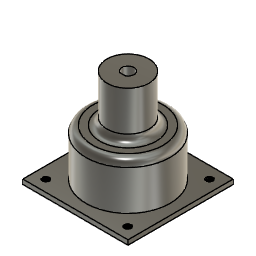
35mm_shaft_extension (Autodesk Fusion 360 design; units mm, degrees)
Autodesk Fusion 360 part; units mm, degrees
sketch "Sketch1" plane through (0, 0, 0) normal (0, 0, 1) x (1, 0, 0)
  line L0 (0, 0) -> (45, 0)
  line L1 (45, 0) -> (45, 45)
  line L2 (45, 45) -> (0, 45)
  line L3 (0, 45) -> (0, 0)
  dimension "d1" = 45
  dimension "d2" = 45
  constraint horizontal L0
  constraint vertical L1
  constraint horizontal L2
  constraint vertical L3
  constraint coincident L0.start L3.end
  measures "d1" distance of L0.start L0.end
  measures "d2" distance of L0.start L2.end
extrude "Extrude1" add sketch "Sketch1" along normal blind 2
sketch "Sketch2" plane through (0, 0, 2) normal (0, 0, 1) x (-1, 0, 0)
  line L0 (0, -45) -> (0, 0)
  line L1 (0, 0) -> (-45, 0)
  line L2 (-45, 0) -> (-45, -45)
  line L3 (-45, -45) -> (0, -45)
  line L4 (-40, -5) -> (-40, -40) construction
  line L5 (-40, -40) -> (-5, -40) construction
  line L6 (-5, -40) -> (-5, -5) construction
  line L7 (-5, -5) -> (-40, -5) construction
  circle A0 centre (-5, -40) radius 1.5
  circle A1 centre (-40, -40) radius 1.5
  circle A2 centre (-5, -5) radius 1.5
  circle A3 centre (-40, -5) radius 1.5
  dimension "d5" = -5
  dimension "d6" = 3
  dimension "d7" = 3
  dimension "d8" = 3
  dimension "d9" = 3
  constraint coincident L5.end L6.start
  constraint coincident L4.end L5.start
  constraint coincident L6.end L7.start
  constraint coincident L4.start L7.end
  measures "d6" diameter of A0
  measures "d7" diameter of A1
  measures "d8" diameter of A2
  measures "d9" diameter of A3
hole "Hole1" at (5, 40, 2) at (40, 40, 2) at (40, 5, 2) at (5, 5, 2) direction (0, 0, -1) diameter 2.529 depth 2 tip angle 118
thread "Thread1" "ISO Metric profile 3.0 M3x0.5 M3x0.5 6H" major diameter 3.086 minor diameter 2.529 pitch 0.5 angle 60 modelled right hand crest width 0.1368 on face at (3.7359, 40.0315, 1.3333) crest through (6.2645, 40, 1.875) on face at (5.1259, 3.7418, 1.3333) crest through (6.2645, 5, 1.875) on face at (40.8128, 40.9687, 1.3333) crest through (41.2645, 40, 1.875) on face at (40.1259, 6.2582, 1.3333) crest through (41.2645, 5, 1.875)
sketch "Sketch3" plane through (0, 0, 2) normal (0, 0, 1) x (-1, 0, 0)
  spline S0 degree 3 poles (-40.9581, -5.8252) (-41.0802, -5.7112) (-41.1784, -5.574) (-41.3207, -5.264) (-41.3611, -5.093) (-41.3757, -4.7382) (-41.3471, -4.5577) (-41.2212, -4.2109) (-41.1226, -4.0488) (-40.9156, -3.8208) (-40.8244, -3.7423) (-40.6232, -3.6071) (-40.5136, -3.5514) (-40.3985, -3.5094) knots 0 0 0 0 0.050111 0.050111 0.102261 0.102261 0.15645 0.15645 0.212677 0.212677 0.24852 0.24852 0.285143 0.285143 0.285143 0.285143
  arc A0 (-39.6015, -3.5094) -> (-40.3985, -3.5094) centre (-40, -5) ccw
  spline S1 degree 3 poles (-39.6015, -3.5094) (-39.4166, -3.5769) (-39.2465, -3.6793) (-38.9611, -3.9399) (-38.8468, -4.0935) (-38.6876, -4.4304) (-38.6419, -4.6092) (-38.6233, -4.9674) (-38.648, -5.1432) (-38.741, -5.4082) (-38.7875, -5.5028) (-38.901, -5.6765) (-38.967, -5.7553) (-39.0419, -5.8252) knots 0 0 0 0 0.059039 0.059039 0.116033 0.116033 0.170983 0.170983 0.223888 0.223888 0.255505 0.255505 0.286347 0.286347 0.286347 0.286347
  arc A1 (-40.9581, -5.8252) -> (-39.0419, -5.8252) centre (-40, -5) ccw
  spline S2 degree 3 poles (-5.9581, -40.8252) (-6.0802, -40.7112) (-6.1784, -40.574) (-6.3207, -40.264) (-6.3611, -40.093) (-6.3757, -39.7382) (-6.3471, -39.5577) (-6.2212, -39.2109) (-6.1226, -39.0488) (-5.9156, -38.8208) (-5.8244, -38.7423) (-5.6232, -38.6071) (-5.5136, -38.5514) (-5.3985, -38.5094) knots 0 0 0 0 0.050111 0.050111 0.102261 0.102261 0.15645 0.15645 0.212677 0.212677 0.24852 0.24852 0.285143 0.285143 0.285143 0.285143
  arc A2 (-4.6015, -38.5094) -> (-5.3985, -38.5094) centre (-5, -40) ccw
  spline S3 degree 3 poles (-4.6015, -38.5094) (-4.4166, -38.5769) (-4.2465, -38.6793) (-3.9611, -38.9399) (-3.8468, -39.0935) (-3.6876, -39.4304) (-3.6419, -39.6092) (-3.6233, -39.9674) (-3.648, -40.1432) (-3.741, -40.4082) (-3.7875, -40.5028) (-3.901, -40.6765) (-3.967, -40.7553) (-4.0419, -40.8252) knots 0 0 0 0 0.059039 0.059039 0.116033 0.116033 0.170983 0.170983 0.223888 0.223888 0.255505 0.255505 0.286347 0.286347 0.286347 0.286347
  arc A3 (-5.9581, -40.8252) -> (-4.0419, -40.8252) centre (-5, -40) ccw
  spline S4 degree 3 poles (-40.9581, -40.8252) (-41.0802, -40.7112) (-41.1784, -40.574) (-41.3207, -40.264) (-41.3611, -40.093) (-41.3757, -39.7382) (-41.3471, -39.5577) (-41.2212, -39.2109) (-41.1226, -39.0488) (-40.9156, -38.8208) (-40.8244, -38.7423) (-40.6232, -38.6071) (-40.5136, -38.5514) (-40.3985, -38.5094) knots 0 0 0 0 0.050111 0.050111 0.102261 0.102261 0.15645 0.15645 0.212677 0.212677 0.24852 0.24852 0.285143 0.285143 0.285143 0.285143
  arc A4 (-39.6015, -38.5094) -> (-40.3985, -38.5094) centre (-40, -40) ccw
  spline S5 degree 3 poles (-39.6015, -38.5094) (-39.4166, -38.5769) (-39.2465, -38.6793) (-38.9611, -38.9399) (-38.8468, -39.0935) (-38.6876, -39.4304) (-38.6419, -39.6092) (-38.6233, -39.9674) (-38.648, -40.1432) (-38.741, -40.4082) (-38.7875, -40.5028) (-38.901, -40.6765) (-38.967, -40.7553) (-39.0419, -40.8252) knots 0 0 0 0 0.059039 0.059039 0.116033 0.116033 0.170983 0.170983 0.223888 0.223888 0.255505 0.255505 0.286347 0.286347 0.286347 0.286347
  arc A5 (-40.9581, -40.8252) -> (-39.0419, -40.8252) centre (-40, -40) ccw
  spline S6 degree 3 poles (-5.9581, -5.8252) (-6.0802, -5.7112) (-6.1784, -5.574) (-6.3207, -5.264) (-6.3611, -5.093) (-6.3757, -4.7382) (-6.3471, -4.5577) (-6.2212, -4.2109) (-6.1226, -4.0488) (-5.9156, -3.8208) (-5.8244, -3.7423) (-5.6232, -3.6071) (-5.5136, -3.5514) (-5.3985, -3.5094) knots 0 0 0 0 0.050111 0.050111 0.102261 0.102261 0.15645 0.15645 0.212677 0.212677 0.24852 0.24852 0.285143 0.285143 0.285143 0.285143
  arc A6 (-4.6015, -3.5094) -> (-5.3985, -3.5094) centre (-5, -5) ccw
  spline S7 degree 3 poles (-4.6015, -3.5094) (-4.4166, -3.5769) (-4.2465, -3.6793) (-3.9611, -3.9399) (-3.8468, -4.0935) (-3.6876, -4.4304) (-3.6419, -4.6092) (-3.6233, -4.9674) (-3.648, -5.1432) (-3.741, -5.4082) (-3.7875, -5.5028) (-3.901, -5.6765) (-3.967, -5.7553) (-4.0419, -5.8252) knots 0 0 0 0 0.059039 0.059039 0.116033 0.116033 0.170983 0.170983 0.223888 0.223888 0.255505 0.255505 0.286347 0.286347 0.286347 0.286347
  arc A7 (-5.9581, -5.8252) -> (-4.0419, -5.8252) centre (-5, -5) ccw
  line L0 (0, -45) -> (0, 0)
  line L1 (0, 0) -> (-45, 0)
  line L2 (-45, 0) -> (-45, -45)
  line L3 (-45, -45) -> (0, -45)
  circle A8 centre (-22.5, -22.5) radius 18
  dimension "d15" = 36
  dimension "d16" = 22.5
  dimension "d17" = 22.5
  measures "d15" diameter of A8
  measures "d16" distance of L2 A8.centre
  measures "d17" distance of L1 A8.centre
extrude "Extrude2" add sketch "Sketch3" along normal blind 20 contours A8
sketch "Sketch4" plane through (0, 0, 22) normal (0, 0, 1) x (-1, 0, 0)
  circle A0 centre (-22.5, -22.5) radius 18
  circle A1 centre (-22.5, -22.5) radius 9
  dimension "d20" = 18
  constraint concentric A0 A1
  measures "d20" diameter of A1
extrude "Extrude3" add sketch "Sketch4" along normal blind 40 contours A1
sketch "Sketch5" plane through (0, 0, 62) normal (0, 0, 1) x (-1, 0, 0)
  circle A0 centre (-22.5, -22.5) radius 9
  line L0 (-21.2668, -20.1827) -> (-23.7332, -20.1827)
  arc A1 (-23.7332, -20.1827) -> (-21.2668, -20.1827) centre (-22.5, -22.5) ccw
  dimension "d23" = 5.25
  constraint concentric A0 A1
  constraint horizontal L0
  measures "d23" diameter of A1
extrude "Extrude4" cut sketch "Sketch5" against normal blind 40 contours L0 A1
fillet "Fillet1" radius 3 2 edges at (30.8909, 19.2455, 22) (39.2819, 29.0091, 22)
extrude "Extrude5" cut 1 faces at (22.2758, 17.9635, 62) along direction (0, 0, -1) blind 20
